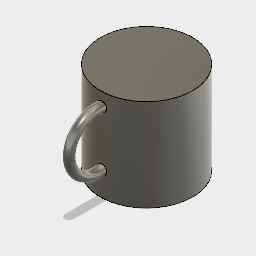
水杯 v1 (Autodesk Fusion 360 design; units mm, degrees)
Autodesk Fusion 360 part; units mm, degrees
cylinder "圆柱体基本要素1" add diameter 20 height 20 placed x (1, 0, 0) y (0, 0, -1) z (0, 1, 0) at (0, 0, 0) makes body 1
cylinder "圆柱体基本要素2" add diameter 18 height 20 placed x (1, 0, 0) y (0, 0, -1) z (0, 1, 0) at (25, 0, 0) separate body makes body 2
torus "圆环体基本要素1" add centre line diameter 12 section diameter 2 placed x (1, 0, 0) y (0, 0, -1) z (0, 1, 0) at (-25, 0, 10) separate body makes body 3
move_body "MoveFace1" bodies 3 to x (0, 1, 0) y (-1, 0, 0) z (0, 0, 1) at (0.2655, 36.2713, 1.0448) on bodies 3
combine "合并1" operation add target body 1 tool bodies 3
move_body "对齐1" bodies 1 to x (1, 0, 0) y (0, 1, 0) z (0, 0, 1) at (25, 0, 0)
move_face "偏移面1" offset -2 1 faces at (23.096, 20, 2.7926) on bodies 2
combine "合并2" operation cut target body 1 tool bodies 2
